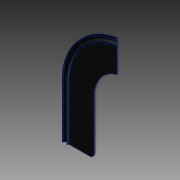
# Autodesk Inventor part: 1122_Middle Heat Sink_V1
Saved by Autodesk Inventor 2020 (Build 240168000, 168)
## iProperties
Created: 2019-07-29
Part Number: 1122_Middle Heat Sink_V1
Material: Aluminum 6061
Document SubType Name: Modeling
Designer: RFLab
Density: 2.7 g/cm^3
Appearance: Aluminum - Flat
Author: RFLab
Autodesk Inventor part; units mm, degrees
ref_plane "YZ Plane" through (0, 0, 0) normal (1, 0, 0) x (0, 1, 0)
ref_plane "XZ Plane" through (0, 0, 0) normal (0, 1, 0) x (-1, 0, 0)
ref_plane "Work Plane1" through (0, 0, 0) normal (0, 0, 1) x (1, 0, 0)
sketch "Sketch1" plane through (0, 0, 0) normal (0, 0, 1) x (1, 0, 0)
  line L0 (-135, 150) -> (-135, -150)
  arc A0 (-135, -150) -> (135, -150) centre (0, -150) ccw
  line L1 (135, -150) -> (135, 150)
  arc A1 (135, 150) -> (-135, 150) centre (0, 150) ccw
  line L2 (-80, -150) -> (-80, 150)
  arc A2 (80, 150) -> (-80, 150) centre (0, 150) ccw
  line L3 (80, 150) -> (80, -150)
  arc A3 (-80, -150) -> (80, -150) centre (0, -150) ccw
  line L4 (0, 0) -> (-135, 0)
  line L5 (0, 0) -> (0, 285)
  line L6 (-75, 150) -> (-75, -150)
  arc A4 (-75, -150) -> (75, -150) centre (0, -150) ccw
  line L7 (75, -150) -> (75, 150)
  arc A5 (75, 150) -> (-75, 150) centre (0, 150) ccw
  point P0 (0, 230)
  point P1 (-80, 0)
  point P2 (0, 225)
  point P3 (-75, 0)
  point P4 (135, 0)
  point P5 (-75, 0)
  point P6 (0, -230)
  dimension "d18" = 5
  dimension "d34" = 300
  dimension "d37" = 55
  dimension "d38" = 75
  dimension "d39" = 75
  constraints: 16 end point, 14 point on circle, 6 centre point, 6 tangent, 5 parallel, 3 horizontal alignment, 3 midpoint, 1 vertical, 1 vertical alignment, 3 other
  measures "d18" distance between parallel lines of L2 L6
  measures "d34" distance of L1.start L1.end
  measures "d37" distance between parallel lines of L0 L2
  measures "d38" radius of A5
  measures "d39" radius of A4
extrude "Extrusion1" add sketch "Sketch1" along normal blind 3 contours A1 L5 A2 L2 L4 L0 | L2 A2 L5 A5 L6 L4
sketch "Sketch2" plane through (0, 0, 3) normal (0, 0, 1) x (1, 0, 0)
  arc A0 (0, 285) -> (-135, 150) centre (0, 150) ccw projected
  line L0 (-135, 150) -> (-135, 0) projected
  line L1 (-135, 0) -> (-75, 0) construction
  line L2 (0, 225) -> (0, 285) construction
  line L3 (-75, 0) -> (-75, 150) projected
  arc A1 (0, 225) -> (-75, 150) centre (0, 150) ccw projected
  point P0 (0, 0)
sketch "Sketch3" plane through (-135, 0, 0) normal (0, -1, 0) x (1, 0, 0)
  line L0 (0, 0) -> (-13, 0)
  line L1 (-13, 0) -> (-13, 6.35)
  line L2 (-13, 6.35) -> (0, 6.35)
  line L3 (0, 6.35) -> (0, 0)
  circle A0 centre (-6.5, 6.35) radius 4.7625 construction
  line L4 (-11.2625, 11.1125) -> (-1.7375, 11.1125)
  line L5 (-1.7375, 11.1125) -> (-1.7375, 1.5875)
  line L6 (-1.7375, 1.5875) -> (-11.2625, 1.5875)
  line L7 (-11.2625, 1.5875) -> (-11.2625, 11.1125)
  line L8 (-11.2625, 11.1125) -> (-1.7375, 1.5875) construction
  line L9 (-1.7375, 11.1125) -> (-11.2625, 1.5875) construction
  point P0 (135, 0)
  point P1 (-1.7375, 6.35)
  point P2 (-11.2625, 6.35)
  point P3 (-1.7375, 6.35)
  point P4 (-11.2625, 6.35)
  dimension "d2" = 13
  dimension "d3" = 6.35
  dimension "d4" = 9.525
  dimension "d5" = 0
  constraints: 20 end point, 4 parallel, 3 midpoint, 2 coincident, 2 horizontal, 2 perpendicular, 1 centre point
  measures "d2" distance of L1.end L2.end
  measures "d3" distance of L0.end L1.end
  measures "d4" diameter of A0
  measures "d5" distance from line of L2 A0.centre
sweep "Sweep1" add profiles "Sketch3" path "Sketch2" path curves L0 A0 contours L0 L1 L2 L7 L6 L5 L3
sketch "Sketch6" plane through (-75, 0, 0) normal (0, -1, 0) x (1, 0, 0)
  arc A0 (-63.7625, 6.35) -> (-54.2375, 6.35) centre (-59, 6.35) ccw projected
  circle A1 centre (-59, 6.35) radius 4.7625
  circle A2 centre (-59, 6.35) radius 3.175
  point P0 (75, 0)
  point P1 (-54.2375, 6.35)
  dimension "d14" = 9.525
  dimension "d15" = 6.35
  constraints: 2 centre point, 2 coincident
  measures "d14" diameter of A1
  measures "d15" diameter of A2
sketch3d "3D Sketch1"
sweep "Sweep2" [suppressed]
sketch "Sketch4" plane through (0, 0, 3) normal (0, 0, 1) x (1, 0, 0)
  line L0 (0, 0) -> (-148.7625, 0)
  line L1 (-148.7625, 0) -> (-148.7625, 20)
  line L2 (-148.7625, 20) -> (0, 20)
  line L3 (0, 20) -> (0, 0)
  line L4 (0, 0) -> (-20, 0)
  line L5 (-20, 0) -> (-20, 308)
  line L6 (-20, 308) -> (0, 308)
  line L7 (0, 308) -> (0, 0)
  line L8 (-138.7625, 0) -> (-138.7625, 300) projected
  point P0 (0, 298)
  point P1 (-20, 20)
  point P2 (-138.7625, 20)
  dimension "d8" = 20
  dimension "d9" = 20
  dimension "d10" = 10
  dimension "d11" = 10
  constraints: 16 end point, 4 parallel, 2 horizontal, 2 perpendicular
  measures "d8" distance of L0.end L1.end
  measures "d9" distance of L5.end L6.end
  measures "d10" distance between parallel lines of L8 L1
  measures "d11" distance from line of point (0, 298) L6
extrude "Extrusion2" cut sketch "Sketch4" against normal through all both and the other way through all contours L0 L8 L2 L5 | L2 L5 L6 L7 | L0 L1 L2 L8 bodies 1
sketch "Sketch7" plane through (0, 0, 3) normal (0, 0, 1) x (1, 0, 0)
  line L0 (-20, 222.2842) -> (-20, 283.5103) projected
  arc A0 (-20, 283.5103) -> (-135, 150) centre (0, 150) ccw projected
  line L1 (-135, 150) -> (-135, 0) projected
  line L2 (-135, 20) -> (-75, 20) projected
  line L3 (-75, 20) -> (-75, 150) projected
  arc A1 (-20, 222.2842) -> (-75, 150) centre (0, 150) ccw projected
  line L4 (-78.5, 150) -> (-78.5, 23.5)
  line L5 (-78.5, 23.5) -> (-131.5, 23.5)
  line L6 (-131.5, 23.5) -> (-131.5, 150)
  arc A2 (-23.5, 279.3832) -> (-131.5, 150) centre (0, 150) ccw
  line L7 (-23.5, 279.3832) -> (-23.5, 224.8999)
  arc A3 (-23.5, 224.8999) -> (-78.5, 150) centre (0, 150) ccw
  point P0 (0, 0)
  point P1 (-131.5, 33.5)
  point P2 (-127.5939, 181.8127)
  point P3 (-116.1076, 211.7355)
  point P4 (-97.7235, 237.9907)
  point P5 (-73.5339, 259.0184)
  point P6 (-44.9756, 273.5696)
  point P7 (-131.5, 66.5)
  point P8 (-131.5, 99.5)
  point P9 (-131.5, 132.5)
  dimension "d21" = 3.5
  dimension "d24" = 70
  dimension "d26" = 10
  dimension "d29" = 33
  constraints: 8 end point, 4 point on circle, 2 centre point, 1 coincident, 1 point on line, 1 vertical, 14 other
  measures "d21" distance between parallel lines of L3 L4
  measures "d26" distance of L5.end point (-131.5, 33.5)
  measures "d29" distance of point (-131.5, 33.5) point (-131.5, 66.5)
hole "Hole1" at (-131.5, 33.5, 3) at (-131.5, 150, 3) at (-127.5939, 181.8127, 3) at (-116.1076, 211.7355, 3) at (-97.7235, 237.9907, 3) at (-73.5339, 259.0184, 3) at (-44.9756, 273.5696, 3) at (-131.5, 66.5, 3) at (-131.5, 99.5, 3) at (-131.5, 132.5, 3) direction (0, 0, -1) diameter 3.4 end through all bodies 1
fillet "Fillet1" radius 10 1 edges at (-75, 20, 1.5)
sketch "Sketch8" plane through (0, 0, 3) normal (0, 0, 1) x (1, 0, 0)
  arc A0 (-85, 20) -> (-75, 30) centre (-85, 30) ccw projected
  line L0 (-75, 30) -> (-75, 150) projected
  arc A1 (-20, 222.2842) -> (-75, 150) centre (0, 150) ccw projected
  line L1 (-20, 222.2842) -> (-20, 283.5103) projected
  arc A2 (-20, 283.5103) -> (-135, 150) centre (0, 150) ccw projected
  line L2 (-135, 150) -> (-135, 20) projected
  line L3 (-135, 20) -> (-85, 20) projected
  line L4 (-74.9, 150) -> (-74.9, 30)
  arc A3 (-85, 19.9) -> (-74.9, 30) centre (-85, 30) ccw
  line L5 (-85, 19.9) -> (-135.1, 19.9)
  line L6 (-135.1, 19.9) -> (-135.1, 150)
  arc A4 (-19.9, 283.6263) -> (-135.1, 150) centre (0, 150) ccw
  line L7 (-19.9, 283.6263) -> (-19.9, 222.208)
  arc A5 (-19.9, 222.208) -> (-74.9, 150) centre (0, 150) ccw
  point P0 (0, 0)
  dimension "d48" = 0.1
  constraints: 8 end point, 6 point on circle, 3 centre point, 6 other
  measures "d48" radial gap between concentric circles of A1 A5
extrude "Extrusion3" [suppressed]
sketch "Sketch11" plane through (0, 0, 3) normal (0, 0, 1) x (1, 0, 0)
  line L0 (-135, 150) -> (-135, 20) projected
  circle A0 centre (-131.5, 99.5) radius 1.7 projected
  circle A1 centre (-44.9756, 273.5696) radius 1.7 projected
  circle A2 centre (-97.7235, 237.9907) radius 1.7 projected
  circle A3 centre (-127.5939, 181.8127) radius 1.7 projected
  circle A4 centre (-131.5, 33.5) radius 1.7 projected
  circle A5 centre (-131.5, 150) radius 1.7 projected
  circle A6 centre (-116.1076, 211.7355) radius 1.7 projected
  circle A7 centre (-73.5339, 259.0184) radius 1.7 projected
  circle A8 centre (-131.5, 66.5) radius 1.7 projected
  circle A9 centre (-131.5, 132.5) radius 1.7 projected
  line L1 (-20, 277.0859) -> (-20, 222.2842)
  arc A10 (-20, 222.2842) -> (-75, 150) centre (0, 150) ccw projected
  arc A11 (-23, 224.5319) -> (-78, 150) centre (0, 150) ccw
  line L2 (-23, 224.5319) -> (-23, 276.5773)
  line L3 (-135, 20) -> (-85, 20) projected
  line L4 (-128.65, 20) -> (-85, 20)
  arc A12 (-85, 20) -> (-75, 30) centre (-85, 30) ccw projected
  arc A13 (-85, 23) -> (-78, 30) centre (-85, 30) ccw
  line L5 (-85, 23) -> (-131.0405, 23)
  line L6 (-78, 150) -> (-78, 30)
  arc A14 (-85, 20) -> (-75, 30) centre (-85, 30) ccw projected
  line L7 (-75, 30) -> (-75, 150) projected
  line L8 (-20, 222.2842) -> (-20, 283.5103) projected
  arc A15 (-20, 283.5103) -> (-135, 150) centre (0, 150) ccw projected
  point P0 (0, 0)
  dimension "d53" = 3
  dimension "d54" = 3
  constraints: 10 end point, 4 point on circle, 2 centre point, 2 horizontal, 2 vertical
  measures "d53" radial gap between concentric circles of A10 A11
  measures "d54" radial gap between concentric circles of A12 A13
sketch "Sketch12" plane through (0, 0, 3) normal (0, 0, 1) x (1, 0, 0)
  arc A0 (-85, 20) -> (-75, 30) centre (-85, 30) ccw projected
  line L0 (-75, 30) -> (-75, 150) projected
  arc A1 (-20, 222.2842) -> (-75, 150) centre (0, 150) ccw projected
  line L1 (-20, 222.2842) -> (-20, 283.5103) projected
  arc A2 (-20, 283.5103) -> (-135, 150) centre (0, 150) ccw projected
  line L2 (-135, 150) -> (-135, 20) projected
  line L3 (-135, 20) -> (-85, 20) projected
  circle A3 centre (-131.5, 99.5) radius 1.7 projected
  circle A4 centre (-44.9756, 273.5696) radius 1.7 projected
  circle A5 centre (-97.7235, 237.9907) radius 1.7 projected
  circle A6 centre (-127.5939, 181.8127) radius 1.7 projected
  circle A7 centre (-131.5, 33.5) radius 1.7 projected
  circle A8 centre (-131.5, 150) radius 1.7 projected
  circle A9 centre (-116.1076, 211.7355) radius 1.7 projected
  circle A10 centre (-73.5339, 259.0184) radius 1.7 projected
  circle A11 centre (-131.5, 66.5) radius 1.7 projected
  circle A12 centre (-131.5, 132.5) radius 1.7 projected
  point P0 (0, 0)
  point P1 (-106.1535, 4.76)
  point P2 (-134.9295, 287.3233)
  dimension "d55" = 15.24
  measures "d55" distance from line of L3 point (-106.153, 4.76)
fillet "Fillet2" radius 4.7625 4 edges at (-110.2678, 246.0923, 1.5875) (-146.2625, 85, 1.5875) (-103.5179, 239.3375, 1.5875) (-136.7375, 85, 1.5875)
equation "\"d39\" = d38"
body "Solid1"
body "Solid2"
